3d printing plate_v2 (Autodesk Fusion 360 design; units mm, degrees)
Autodesk Fusion 360 part; units mm, degrees
sketch "Sketch1" plane through (0, 0, 0) normal (0, 1, 0) x (1, 0, 0)
  line L0 (120, -5) -> (120, -70)
  line L1 (0, -70) -> (0, -5)
  circle A0 centre (12, -30) radius 3
  circle A1 centre (12, -57) radius 3
  circle A2 centre (108, -30) radius 3
  circle A3 centre (108, -57) radius 3
  circle A4 centre (22.5, -43.5) radius 5
  circle A5 centre (97.5, -43.5) radius 5
  line L2 (12, -30) -> (108, -30) construction
  line L3 (108, -30) -> (108, -57) construction
  line L4 (108, -57) -> (12, -57) construction
  line L5 (12, -57) -> (12, -30) construction
  line L6 (12, -35) -> (108, -35)
  line L7 (108, -35) -> (108, -52)
  line L8 (108, -52) -> (12, -52)
  line L9 (12, -52) -> (12, -35)
  line L10 (0, -5) -> (120, -5)
  line L11 (0, -70) -> (0, -75)
  line L12 (0, -75) -> (120, -75)
  line L13 (120, -75) -> (120, -70)
  dimension "d3" = 6
  dimension "d4" = 6
  dimension "d7" = 12
  dimension "d8" = 12
  dimension "d9" = 6
  dimension "d10" = 6
  dimension "d11" = 12
  dimension "d12" = 12
  dimension "d15" = 10
  dimension "d16" = 10
  dimension "d17" = 10.5
  dimension "d18" = 13.5
  dimension "d19" = 13.5
  dimension "d20" = 10.5
  dimension "d23" = 5
  dimension "d24" = 5
  dimension "d36" = 25
  dimension "d37" = 5
  constraint vertical L0
  constraint vertical L1
  constraint coincident A0.centre L2.start
  constraint coincident A2.centre L2.end
  constraint coincident A3.centre L3.end
  constraint coincident A1.centre L4.end
  constraint horizontal L6
  constraint vertical L7
  constraint horizontal L8
  constraint vertical L9
  constraint coincident L3 L7.end
  constraint coincident L5 L6.start
  constraint perpendicular L0 L10
  constraint perpendicular L1 L12
  measures "d3" diameter of A0
  measures "d4" diameter of A1
  measures "d7" distance of L1 A1.centre
  measures "d8" distance of L1 A0.centre
  measures "d9" diameter of A2
  measures "d10" diameter of A3
  measures "d11" distance of L0 A2.centre
  measures "d12" distance of L0 A3.centre
  measures "d15" diameter of A4
  measures "d16" diameter of A5
  measures "d17" distance of A4.centre L5
  measures "d18" distance of A4.centre L2
  measures "d19" distance of A5.centre L2
  measures "d20" distance of A5.centre L3
  measures "d23" distance of A0.centre L6
  measures "d24" distance of A1.centre L8
  measures "d36" distance of A0.centre L10
  measures "d37" distance of L1.start L11.end
extrude "Extrude2" add sketch "Sketch1" along normal blind 10 contours L0 L1 L10 L11 L12 L13 makes body 1
extrude "Extrude3" add sketch "Sketch1" against normal blind 1 separate body contours L6 L7 L8 L9 makes body 2
extrude "Extrude4" add sketch "Sketch1" along normal blind 3 and the other way blind 1 contours A4 | A5 bodies 2
extrude "Extrude5" add sketch "Sketch1" along normal blind 6 contours L6 L7 L8 L9 bodies 1 2
sketch "Sketch2" plane through (0, 6, 0) normal (0, 1, 0) x (-1, 0, 0)
  circle A0 centre (-108, 57) radius 3
  circle A1 centre (-12, 30) radius 3
  circle A2 centre (-12, 57) radius 3
  circle A3 centre (-108, 30) radius 3
  line L0 (-120, 75) -> (-120, 5)
  line L1 (0, 5) -> (0, 75)
  line L2 (0, 75) -> (-120, 75)
  line L3 (-120, 5) -> (0, 5)
  line L4 (-108, 52) -> (-12, 52)
  line L5 (-12, 52) -> (-12, 35)
  line L6 (-12, 35) -> (-108, 35)
  line L7 (-108, 35) -> (-108, 52)
extrude "Extrude6" add 1 faces at (13.8333, 6, 43.5) along direction (0, 1, 0) blind 4 on bodies 1 bodies 1
sketch "Sketch3" plane through (0, 10, 0) normal (0, 1, 0) x (-1, 0, 0)
  circle A0 centre (-22.5, 43.5) radius 5
  circle A1 centre (-97.5, 43.5) radius 5
  circle A2 centre (-12, 57) radius 3
  circle A3 centre (-108, 57) radius 3
  circle A4 centre (-108, 30) radius 3
  circle A5 centre (-12, 30) radius 3
  line L0 (0, 5) -> (0, 75)
  line L1 (0, 75) -> (-120, 75)
  line L2 (-120, 75) -> (-120, 5)
  line L3 (-120, 5) -> (0, 5)
  circle A6 centre (-60, 30) radius 9.5
  line L4 (-12, 30) -> (-108, 30) construction
  circle A7 centre (-60, 30) radius 5
  dimension "d40" = 19
  dimension "d41" = 10
  constraint coincident A5.centre L4.start
  constraint coincident A4.centre L4.end
  constraint midpoint A6.centre L4
  constraint concentric A6 A7
  measures "d40" diameter of A6
  measures "d41" diameter of A7
extrude "Extrude7" cut sketch "Sketch3" against normal blind 20 contours A7 bodies 1
extrude "Extrude8" cut sketch "Sketch3" against normal blind 6 contours A6 bodies 1
